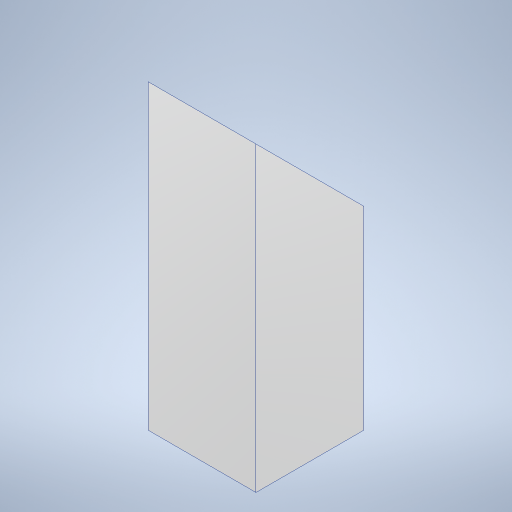
# Autodesk Inventor part: FRONT FRAME RISER
Saved by Autodesk Inventor 2023 (Build 270158000, 158)
## iProperties
Created: 2022-08-25
Part Number: FRONT FRAME RISER
Material: Aluminum 6061
Document SubType Name: Modeling
Designer: D.C. Eksteen
Density: 2.7 g/cm^3
Appearance: Aluminum - Flat
Author: D.C. Eksteen
Title: FRONT FRONT FRAME RISER
Autodesk Inventor part; units mm, degrees
ref_plane "YZ Plane" through (0, 0, 0) normal (1, 0, 0) x (0, 1, 0)
ref_plane "XZ Plane" through (0, 0, 0) normal (0, 1, 0) x (-1, 0, 0)
ref_plane "XY Plane" through (0, 0, 0) normal (0, 0, 1) x (1, 0, 0)
sketch "Sketch1" plane through (0, 0, 0) normal (0, 1, 0) x (-1, 0, 0)
  line L0 (0, 0) -> (25, 0)
  line L1 (25, 0) -> (25, 25)
  line L2 (25, 25) -> (0, 25)
  line L3 (0, 25) -> (0, 0)
  line L4 (22, 22) -> (22, 3)
  line L5 (22, 3) -> (3, 3)
  line L6 (3, 3) -> (3, 22)
  line L7 (3, 22) -> (22, 22)
  dimension "d0" = 25
  dimension "d1" = 25
  dimension "d2" = 3
  constraints: 16 end point, 4 parallel, 2 perpendicular, 1 horizontal, 3 other
  measures "d0" distance of L2.end L1.end
  measures "d1" distance of L1.end L0.end
  measures "d2" distance between parallel lines of L1 L4
extrude "Extrusion1" add sketch "Sketch1" along normal blind 167.25
sketch "Sketch4" plane through (0, 0, 25) normal (1, 0, 0) x (0, 0, -1)
  line L0 (0, 0) -> (25, 0) projected
  line L1 (25, 0) -> (25, 167.25) projected
  line L2 (0, 167.25) -> (25, 167.25) projected
  line L3 (0, 0) -> (0, 167.25) projected
  line L4 (0, 167.25) -> (25, 142.25)
  line L5 (0, 167.25) -> (35.3553, 167.25) construction
  line L6 (0, 167.25) -> (0, 97.25)
  line L7 (0, 0) -> (0, 167.25) projected
  line L8 (0, 97.25) -> (25, 97.25)
  line L9 (25, 142.25) -> (25, 97.25)
  dimension "d12" = 45
  dimension "d13" = 70
  constraints: 10 end point, 3 point on line, 1 collinear, 1 equal length, 1 horizontal, 1 perpendicular
  measures "d12" angle of L4 L5
  measures "d13" distance of L2.start L6.end
extrude "Extrusion4" cut sketch "Sketch4" against normal through all contours L3 L8 L1 L0 | L2 L1 L4
body "Solid1"
